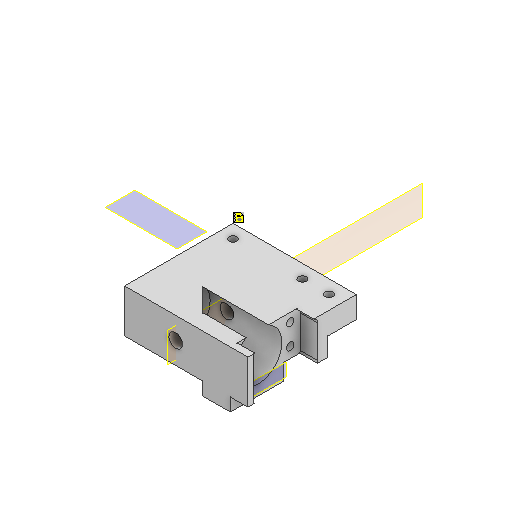
# Autodesk Inventor part: 30_Lightsheet_generator_passive_base_v1
Saved by Autodesk Inventor 2025.3 (Build 293356000, 356)
## iProperties
Created: 2022-12-16
Part Number: 30_Lightsheet_generator_passive_base_v1
Material: Generisch
Document SubType Name: Modeling
Designer: UC2
Density: 1 g/cm^3
Appearance: Vorgabe
Author: UC2
Autodesk Inventor part; units mm, degrees
ref_plane "YZ Plane" through (0, 0, 0) normal (1, 0, 0) x (0, 1, 0)
ref_plane "XZ Plane" through (0, 0, 0) normal (0, 1, 0) x (-1, 0, 0)
ref_plane "XY Plane" through (0, 0, 0) normal (0, 0, 1) x (1, 0, 0)
ref_plane "Arbeitsebene6" through (-62.1, 3.95, -31.1) normal (0, -1, 0) x (1, 0, 0)
sketch "Skizze13" plane through (18.9, 3.95, -31.1) normal (0, 1, 0) x (-1, 0, 0)
  circle A0 centre (40.5, 5) radius 1.45 projected
  line L0 (29.1796, 0.9) -> (29.1796, 0) projected
  line L1 (45.5, 0) -> (29.1796, 0) projected
  line L2 (45.5, 0) -> (45.5, 10) projected
  line L3 (45.5, 10) -> (29.1796, 10) projected
  line L4 (29.1796, 10) -> (29.1796, 6.8717) projected
  line L5 (29.1796, 6.8717) -> (32.9296, 6.8717) projected
  line L6 (32.9296, 6.8717) -> (32.9296, 0.9) projected
  line L7 (32.9296, 0.9) -> (29.1796, 0.9) projected
  line L8 (24.1796, 0) -> (24.1796, 0.9) projected
  line L9 (24.1796, 0.9) -> (20.4296, 0.9) projected
  line L10 (20.4296, 0.9) -> (20.4296, 6.8717) projected
  line L11 (20.4296, 6.8717) -> (24.1796, 6.8717) projected
  line L12 (24.1796, 6.8717) -> (24.1796, 10) projected
  line L13 (24.1796, 10) -> (0, 10) projected
  line L14 (0, 0) -> (0, 10) projected
  line L15 (24.1796, 0) -> (0, 0) projected
  circle A1 centre (14.9199, 5) radius 1.45 projected
  circle A2 centre (5.0801, 5) radius 1.45 projected
  line L16 (29.1796, 10) -> (24.1796, 10)
  line L17 (29.1796, 0) -> (24.1796, 0)
  line L18 (55.5, 0) -> (55.5, 10) projected
  line L19 (55.5, 10) -> (55.473, 10) projected
  line L20 (55.473, 10) -> (55.473, 40) projected
  line L21 (55.473, 40) -> (45.5, 40) projected
  line L22 (45.5, 40) -> (45.5, 20) projected
  line L23 (45.5, 20) -> (35.5, 20) projected
  line L24 (35.5, 20) -> (35.5, 10.0274) projected
  arc A3 (35.5, 10.0274) -> (35.527, 10) centre (40.5, 14.9264) ccw projected
  line L25 (45.5, 10) -> (35.527, 10) projected
  line L26 (45.5, 0) -> (45.5, 10) projected
  line L27 (45.5, 0) -> (55.5, 0) projected
  line L28 (52.073, 16.5) -> (52.073, 3.5) projected
  arc A4 (48.873, 3.5) -> (52.073, 3.5) centre (50.473, 3.5) ccw projected
  line L29 (48.873, 3.5) -> (48.873, 16.5) projected
  arc A5 (52.073, 16.5) -> (48.873, 16.5) centre (50.473, 16.5) ccw projected
  line L30 (48.8865, 23.1111) -> (48.8865, 36.1111) projected
  arc A6 (52.0865, 36.1111) -> (48.8865, 36.1111) centre (50.4865, 36.1111) ccw projected
  line L31 (52.0865, 36.1111) -> (52.0865, 23.1111) projected
  arc A7 (48.8865, 23.1111) -> (52.0865, 23.1111) centre (50.4865, 23.1111) ccw projected
  line L32 (-10, 0) -> (0, 0) projected
  line L33 (0, 10) -> (0, 0) projected
  line L34 (16, 10) -> (0, 10) projected
  line L35 (16, 10) -> (16, 20) projected
  line L36 (16, 20) -> (-10, 20) projected
  line L37 (-10, 20) -> (-10, 0) projected
  line L38 (-3.4, 16.5) -> (-3.4, 3.5) projected
  arc A8 (-6.6, 3.5) -> (-3.4, 3.5) centre (-5, 3.5) ccw projected
  line L39 (-6.6, 3.5) -> (-6.6, 16.5) projected
  arc A9 (-3.4, 16.5) -> (-6.6, 16.5) centre (-5, 16.5) ccw projected
  line L40 (0, 40) -> (45.5, 40)
  line L41 (45.5, 40) -> (45.5, 20.5)
  line L42 (45.5, 20.5) -> (0, 20.5)
  line L43 (0, 20.5) -> (0, 40)
  line L44 (45.5, 20.5) -> (35.5, 20.5)
  line L45 (35.5, 20.5) -> (35.5, 20)
  line L46 (35.5, 20) -> (45.5, 20)
  line L47 (45.5, 20) -> (45.5, 20.5)
  line L48 (16, 20) -> (0, 20)
  line L49 (0, 20) -> (0, 20.5)
  line L50 (0, 20.5) -> (16, 20.5)
  line L51 (16, 20.5) -> (16, 20)
  line L52 (0, 20) -> (0, 10)
  line L53 (35.5, 10) -> (45.5, 10)
  line L54 (45.5, 10) -> (45.5, 20.5)
  line L55 (45.5, 20.5) -> (35.5, 20.5)
  line L56 (35.5, 20.5) -> (35.5, 10)
  line L57 (0, 20.5) -> (-10.5, 20.5)
  line L58 (-10.5, 20.5) -> (-10.5, 0.5)
  line L59 (-10.5, 0.5) -> (0, 0.5)
  line L60 (0, 0.5) -> (0, 20.5)
  point P0 (0, 20)
  point P1 (0.5252, 10)
  point P2 (35.527, 10)
  point P3 (0, 20)
  point P4 (35.5, 10.0274)
  point P5 (-10.5, 20.5)
  dimension "d60" = 0.5
  dimension "d93" = 20
  dimension "d94" = 0.5
  constraints: 47 end point, 11 parallel, 6 horizontal, 6 perpendicular, 2 point on line
  measures "d60" distance between parallel lines of L23 L42
  measures "d93" distance of L57.end L58.end
  measures "d94" distance between parallel lines of L58 L37
extrude "Extrusion12" add sketch "Skizze13" along normal blind 8 contours L7 L6 L5 L4 L3 L2 L1 L0 | L0 L17 L8 L9 L10 L11 L12 L16 L4 L5 L6 L7 | L15 L14 L13 L12 L11 L10 L9 L8 | L3 A3 L24 L23 L54 | L23 L45 L42 L22 | L16 L13 L35 L51 L42 L45 L24 L56 L3 | L42 L43 L40 L22 | L52 L36 L35 L13 | L49 L42 L51 L36
sketch "Skizze16" plane through (18.9, 3.95, -31.1) normal (0, -1, 0) x (1, 0, 0)
  line L0 (-45.5, 0) -> (-45.5, 40) projected
  circle A0 centre (-5.0801, 5) radius 1.45 projected
  circle A1 centre (-14.9199, 5) radius 1.45 projected
  line L1 (-16, 20) -> (10, 20) projected
  line L2 (-66.9798, -10.3003) -> (9.2505, 65.9301)
  line L3 (7.6336, 20.5) -> (0, 20.5) projected
  line L4 (7.6336, 20.5) -> (-54.1544, 20.5)
  line L5 (-54.1544, 20.5) -> (-54.1544, 40)
  line L6 (-54.1544, 40) -> (7.6336, 40)
  line L7 (7.6336, 40) -> (7.6336, 20.5)
  line L8 (-45.5, 40) -> (0, 40) projected
  line L9 (0, 0) -> (-45.5, 0) projected
  line L10 (0, 40) -> (0, 0) projected
  line L11 (0, 40) -> (0, 20.5)
  point P0 (-18.9, 31.1)
  point P1 (-45.5, 20.5)
  point P2 (-45.2879, 40)
  point P3 (10.5, 20.5)
  point P4 (0, 20.5)
  point P5 (0, 40)
  constraints: 12 end point, 2 parallel, 1 horizontal, 1 perpendicular, 1 vertical, 3 other
extrude "Extrusion13" add sketch "Skizze16" along normal blind 8 contours L0 L6 L2 L4 | L2 L6 L10 L4
ref_plane "Arbeitsebene7" through (-7.7796, -1.85, -37.9251) normal (1, 0, 0) x (0, -1, 0)
sketch "Skizze18" plane through (-7.7796, -1.85, -37.9251) normal (1, 0, 0) x (0, -1, 0)
  arc A0 (-5.8, -13.6968) -> (-0.7, -9.8391) centre (-5.8, -8.3968) ccw projected
  line L0 (-0.7, -9.8391) -> (-0.7, -7.7251) projected
  arc A1 (-10.8, -9.8251) -> (-0.8, -9.8251) centre (-5.8, -8.3968) ccw projected
  line L1 (-0.8, -7.8251) -> (-0.8, -9.8251) projected
  line L2 (-10.8, -7.8251) -> (-0.8, -7.8251) projected
  line L3 (-10.8, -9.8251) -> (-10.8, -7.8251) projected
  arc A2 (-10.9, -9.8391) -> (-0.7, -9.8391) centre (-5.8, -8.3968) ccw
  line L4 (-10.9, -9.8391) -> (-10.9, -7.7251)
  line L5 (-10.9, -7.7251) -> (-0.7, -7.7251)
  line L6 (-0.7, -7.7251) -> (-0.7, -9.8391)
  point P0 (-1.85, -37.9251)
  point P1 (-5.8, -13.6968)
  constraints: 6 end point, 2 point on circle, 1 centre point, 3 other
extrude "Extrusion15" cut sketch "Skizze18" along normal mid plane 12.5 contours A2 L4 L5 L0 A0 | L3 L2 L1 A1
ref_plane "Arbeitsebene8" through (22.1204, -2.15, -7.2) normal (1, 0, 0) x (0, 1, 0)
ref_plane "Arbeitsebene9" through (-36.7921, -9.8415, -30.1125) normal (-0.7071068, 0, 0.7071068) x (0.7071068, 0, 0.7071068)
ref_plane "Arbeitsebene10" through (16.1879, 11.05, 2.9992) normal (-1, 0, 0) x (0, 0, 1)
sketch "Skizze21" plane through (16.1879, 11.05, 2.9992) normal (-1, 0, 0) x (0, 0, 1)
  arc A0 (-3.1969, -9.9981) -> (-5.2274, -9.9178) centre (-4.0992, -7.1) ccw projected
  circle A1 centre (-4.0992, -7.1) radius 9
  line L0 (-13.0992, -7.1) -> (4.9008, -7.1)
  line L1 (4.9008, -7.1) -> (4.9008, -20.07)
  line L2 (4.9008, -20.07) -> (-13.0992, -20.07)
  line L3 (-13.0992, -20.07) -> (-13.0992, -7.1)
  point P0 (-2.9992, -11.05)
  dimension "d75" = 18
  constraints: 8 end point, 2 parallel, 2 point on circle, 1 centre point, 1 coincident, 1 horizontal, 1 perpendicular
  measures "d75" diameter of A1
ref_plane "Arbeitsebene11" through (-36.7921, -9.8415, -30.1125) normal (-0.7071068, 0, 0.7071068) x (0.7071068, 0, 0.7071068)
extrude "Extrusion18" cut sketch "Skizze21" along normal up to surface contours L0 A0 | L0 A1 | A0 L0 A1 surface through (-36.7921, -9.8415, -30.1125) normal (-0.7071068, 0, 0.7071068)
sketch "Skizze22" plane through (18.9, -4.05, -31.1) normal (0, -1, 0) x (1, 0, 0)
  line L0 (-34.6684, 23.7083) -> (-19.8191, 38.5575)
  line L1 (-19.8191, 38.5575) -> (-18.9706, 37.709)
  line L2 (-18.9706, 37.709) -> (-33.8198, 22.8597)
  line L3 (-33.8198, 22.8597) -> (-34.6684, 23.7083)
  line L4 (-34.6684, 23.7083) -> (-18.9706, 37.709) construction
  line L5 (-19.8191, 38.5575) -> (-33.8198, 22.8597) construction
  line L6 (-34.6684, 23.7083) -> (-13.6684, 23.7083) construction
  line L7 (-45.5, 40) -> (-45.5, 20.5) projected
  line L8 (0, 40) -> (-45.5, 40) projected
  line L9 (-45.5, 20.5) -> (0, 20.5) projected
  line L10 (0, 20.5) -> (0, 40) projected
  point P0 (-18.9, 31.1)
  point P1 (-26.8195, 30.7086)
  dimension "d78" = 21
  dimension "d79" = 45
  dimension "d80" = 1.2
  constraints: 14 end point, 2 midpoint, 2 parallel, 1 equal length, 1 horizontal, 1 perpendicular
  measures "d78" distance of L0.start L0.end
  measures "d79" angle of L6 L0
  measures "d80" distance of L0.end L1.end
extrude "Extrusion19" cut sketch "Skizze22" against normal blind 14 contours L0 L1 L2 L3
sketch "Skizze23" plane through (18.9, -4.05, -31.1) normal (0, -1, 0) x (1, 0, 0)
  line L0 (-35.6796, 21) -> (-32.9713, 23.7083)
  line L1 (-33.3878, 23.2918) -> (-30.8027, 25.8769) projected
  line L2 (-2.7121, 21) -> (-35.6796, 21) projected
  line L3 (-32.9713, 21) -> (-32.9713, 23.7083)
  line L4 (-18.9706, 37.709) -> (-19.9714, 36.7082) projected
  line L5 (-19.9714, 36.7082) -> (-17.0744, 36.7082)
  line L6 (-17.0744, 36.7082) -> (-17.0744, 39)
  line L7 (-18.9706, 37.709) -> (-33.8198, 22.8597) projected
  line L8 (-19.9714, 36.7082) -> (-17.6796, 39)
  line L9 (-17.6796, 39) -> (-17.0744, 39)
  line L10 (-45.5, 40) -> (-45.5, 20.5) projected
  line L11 (0, 40) -> (-45.5, 40) projected
  line L12 (-45.5, 20.5) -> (0, 20.5) projected
  line L13 (0, 20.5) -> (0, 40) projected
  point P0 (-18.9, 31.1)
  point P1 (-29.1796, 21)
  constraints: 12 end point, 2 horizontal, 2 perpendicular, 2 point on line, 1 collinear
extrude "Extrusion20" add sketch "Skizze23" against normal up to surface (16 mm away) contours L0 L3 L2 | L8 L9 L6 L5 L4
ref_plane "Arbeitsebene12" through (-26.6, -8.85, -11.1) normal (1, 0, 0) x (0, 1, 0)
sketch "Skizze25" plane through (18.9, 3.95, -10.6) normal (1, 0, 0) x (0, 0, -1)
  line L0 (0.5, -6.8) -> (20.5, -6.8) projected
  line L1 (0, -8) -> (0, 8) projected
  line L2 (0, 0) -> (10.5, 0) projected
  line L3 (0, 0) -> (10, 0)
  line L4 (10, 0) -> (10, -6.8)
  line L5 (10, -6.8) -> (0, -6.8)
  line L6 (0, -6.8) -> (0, 0)
  line L7 (10.5, 0) -> (10.5, -6.8) projected
  point P0 (-10.6, -3.95)
  point P1 (0, -6.8)
  dimension "d87" = 0.5
  constraints: 8 end point, 2 parallel, 1 horizontal, 1 perpendicular, 1 point on line
  measures "d87" distance between parallel lines of L7 L4
extrude "Extrusion22" add sketch "Skizze25" against normal up to surface (45.5 mm away) contours L5 L1 L2 L4 L0
sketch "Skizze26" plane through (18.9, 11.95, -31.1) normal (0, 0, -1) x (-1, 0, 0)
  line L0 (0, -8) -> (24.1796, -8) projected
  line L1 (0, 0) -> (24.1796, 0) projected
  line L2 (0, -8) -> (0, 0) projected
  line L3 (24.1796, -8) -> (29.1796, -8) projected
  circle A0 centre (26.6796, -8) radius 2.5
  line L4 (24.1796, -8) -> (24.1796, 0) projected
  point P0 (18.9, -11.95)
  constraints: 1 horizontal alignment, 2 other
extrude "Extrusion23" cut sketch "Skizze26" against normal through all contours A0 L3 | L3 A0
sketch "Skizze30" plane through (-7.7796, -1.85, -37.9251) normal (1, 0, 0) x (0, -1, 0)
  circle A0 centre (-5.8, -38.5222) radius 2.5 projected
  line L0 (-23.3912, -36.8251) -> (18.065, -36.8251)
  circle A1 centre (-5.8, -36.8251) radius 0.9537
  point P0 (-1.85, -37.9251)
  constraints: 2 end point, 1 centre point, 1 horizontal, 1 point on line, 2 other
extrude "Extrusion27" cut sketch "Skizze30" against normal blind 12 contours A1 L0 A0 | A0 A1 | A1 L0 picked at (-5.7305, -36.5604)
sketch "Skizze31" plane through (18.9, 3.95, -31.1) normal (1, 0, 0) x (0, 0, -1)
  arc A0 (-23, -8) -> (-22, -7) centre (-23, -7) ccw projected
  line L0 (-22, 7) -> (-22, -7) projected
  arc A1 (-22, 7) -> (-23, 8) centre (-23, 7) ccw projected
  line L1 (-37, 8) -> (-23, 8) projected
  arc A2 (-37, 8) -> (-38, 7) centre (-37, 7) ccw projected
  line L2 (-38, -7) -> (-38, 7) projected
  arc A3 (-38, -7) -> (-37, -8) centre (-37, -7) ccw projected
  line L3 (-23, -8) -> (-37, -8) projected
  arc A4 (-32.728, 6.725) -> (-34.46, 5.725) centre (-32.728, 4.725) ccw projected
  line L4 (-27.272, 6.725) -> (-32.728, 6.725) projected
  arc A5 (-25.54, 5.725) -> (-27.272, 6.725) centre (-27.272, 4.725) ccw projected
  line L5 (-22.812, 1) -> (-25.54, 5.725) projected
  arc A6 (-22.812, -1) -> (-22.812, 1) centre (-24.544, 0) ccw projected
  line L6 (-25.54, -5.725) -> (-22.812, -1) projected
  arc A7 (-27.272, -6.725) -> (-25.54, -5.725) centre (-27.272, -4.725) ccw projected
  line L7 (-32.728, -6.725) -> (-27.272, -6.725) projected
  arc A8 (-34.46, -5.725) -> (-32.728, -6.725) centre (-32.728, -4.725) ccw projected
  line L8 (-37.188, -1) -> (-34.46, -5.725) projected
  arc A9 (-37.188, 1) -> (-37.188, -1) centre (-35.456, 0) ccw projected
  line L9 (-34.46, 5.725) -> (-37.188, 1) projected
  circle A10 centre (-17.9023, -2.836) radius 1.4 projected
  circle A11 centre (-17.9023, 4.925) radius 1.4 projected
  line L10 (-20.1, -8) -> (-20.1, -6.7) projected
  line L11 (-20.1, -6.7) -> (-14.4396, -6.7) projected
  arc A12 (-14.4396, -6.7) -> (-14.3131, -6) centre (-16.3131, -6) ccw projected
  line L12 (-14.3131, -6) -> (-14.3131, 6) projected
  arc A13 (-14.3131, 6) -> (-16.3131, 8) centre (-16.3131, 6) ccw projected
  line L13 (-16.3131, 8) -> (-23, 8) projected
  arc A14 (-22, 7) -> (-23, 8) centre (-23, 7) ccw projected
  line L14 (-22, -7) -> (-22, 7) projected
  arc A15 (-23, -8) -> (-22, -7) centre (-23, -7) ccw projected
  line L15 (-23, -8) -> (-20.1, -8) projected
  line L16 (-23, 8.1) -> (-16.3131, 8.1)
  arc A16 (-14.2131, 6) -> (-16.3131, 8.1) centre (-16.3131, 6) ccw
  line L17 (-14.2131, 6) -> (-14.2131, -6)
  arc A17 (-14.3715, -6.8) -> (-14.2131, -6) centre (-16.3131, -6) ccw
  line L18 (-14.3715, -6.8) -> (-20, -6.8)
  line L19 (-20, -6.8) -> (-20, -8.1)
  line L20 (-20, -8.1) -> (-23, -8.1)
  line L21 (-23, -8.1) -> (-37, -8.1)
  arc A18 (-38.1, -7) -> (-37, -8.1) centre (-37, -7) ccw
  line L22 (-38.1, -7) -> (-38.1, 7)
  arc A19 (-37, 8.1) -> (-38.1, 7) centre (-37, 7) ccw
  line L23 (-37, 8.1) -> (-23, 8.1)
  point P0 (-31.1, -3.95)
  dimension "d113" = 0.1
  dimension "d114" = 0.1
  constraints: 16 end point, 8 point on circle, 4 centre point, 10 other
  measures "d113" distance between parallel lines of L11 L18
  measures "d114" distance between parallel lines of L3 L21
ref_plane "Arbeitsebene13" through (12.4, -4.05, -16.7869) normal (-1, 0, 0) x (0, 0, 1)
extrude "Extrusion28" cut sketch "Skizze31" against normal up to surface (6.5 mm away) contours L3 A3 L2 A2 L1 A1 L0 A0 | A0 L0 A1 L13 A13 L12 A12 L11 L10 L15 | L4 A5 L5 A6 L6 A7 L7 A8 L8 A9 L9 A4 | A10 | A11 | L16 A16 L17 A17 L18 L19 L20 L21 A18 L22 A19 L23
sketch "Skizze32" plane through (12.4, -2.05, -16.7869) normal (1, 0, 0) x (0, 0, -1)
  circle A0 centre (-3.5892, 3.164) radius 1.4 projected
  circle A1 centre (-3.5892, 10.925) radius 1.4 projected
  point P0 (-16.7869, 2.05)
extrude "Extrusion29" cut sketch "Skizze32" against normal blind 10
sketch "Skizze33" plane through (12.4, -3.05, 7) normal (1, 0, 0) x (0, 0, -1)
  line L0 (38.1, -5.8) -> (18.1, -5.8) projected
  line L1 (38.1, -5.8) -> (38.1, 0.2) projected
  line L2 (18.1, 0.2) -> (38.1, 0.2) projected
  line L3 (18.1, -5.8) -> (18.1, 0.2) projected
  line L4 (15.1, -1) -> (18, -1) projected
  line L5 (0.6417, -1) -> (-1.9, -1) projected
  line L6 (17.6, 0.2) -> (17.6, -1) projected
  line L7 (15.1, -1) -> (1.1, -1) projected
  arc A0 (12.2231, -1) -> (12.2231, 15) centre (8.1, 7) ccw projected
  circle A1 centre (8.1, 7) radius 9
  line L8 (17.6, -1) -> (17.6, -5.8)
  line L9 (17.6, -5.8) -> (-1.9, -5.8)
  line L10 (-1.9, -5.8) -> (-1.9, -1)
  line L11 (-1.9, -1) -> (17.6, -1) projected
  line L12 (3.9769, -1) -> (-1.9, -1)
  point P0 (7, 3.05)
  point P1 (3.9769, -1)
  constraints: 8 end point, 2 perpendicular, 2 point on circle, 1 centre point, 1 coincident, 1 horizontal, 1 point on line, 1 vertical
ref_plane "Arbeitsebene14" through (-36.7921, -9.8415, -30.1125) normal (-0.7071068, 0, 0.7071068) x (0.7071068, 0, 0.7071068)
extrude "Extrusion30" add sketch "Skizze33" against normal up to surface contours L4 L8 L9 L10 L5 L11 L7 A1 surface through (-36.7921, -9.8415, -30.1125) normal (-0.7071068, 0, 0.7071068)
sketch "Skizze34" plane through (12.4, -8.85, -10.6) normal (0, -1, 0) x (1, 0, 0)
  line L0 (-12.4706, 17.209) -> (-13.4714, 16.2082) projected
  line L1 (-13.3191, 18.0575) -> (-12.4706, 17.209) projected
  line L2 (-28.1684, 3.2083) -> (-13.3191, 18.0575) projected
  line L3 (-27.3198, 2.3597) -> (-28.1684, 3.2083) projected
  line L4 (-26.4713, 3.2083) -> (-27.3198, 2.3597) projected
  line L5 (-13.4714, 16.2082) -> (-26.4713, 3.2083) projected
  line L6 (-13.3191, 18.4897) -> (-12.0384, 17.209)
  line L7 (-12.0384, 17.209) -> (-13.2553, 15.9921)
  line L8 (-13.2553, 15.9921) -> (-26.2552, 2.9922)
  line L9 (-26.2552, 2.9922) -> (-27.3198, 1.9276)
  line L10 (-27.3198, 1.9276) -> (-28.6005, 3.2083)
  line L11 (-28.6005, 3.2083) -> (-13.3191, 18.4897)
  point P0 (-12.4, 10.6)
  constraints: 12 end point, 5 other
extrude "Extrusion31" cut sketch "Skizze34" against normal blind 10 contours L0 L5 L4 L3 L2 L1 | L6 L7 L8 L9 L10 L11
sketch "Skizze35" plane through (12.4, -2.05, -16.8869) normal (1, 0, 0) x (0, 0, -1)
  circle A0 centre (-3.6892, 3.164) radius 1.4 projected
  circle A1 centre (-3.6892, 10.925) radius 1.4 projected
  arc A2 (-23.8869, 2.077) -> (-11.6638, 14) centre (-15.7869, 6) ccw projected
  line L0 (-23.8869, 2.077) -> (-23.8869, -1) projected
  arc A3 (-23.8869, -1) -> (-23.2452, -2) centre (-22.7869, -1) ccw projected
  line L1 (-25.7869, -2) -> (-23.2452, -2) projected
  line L2 (-25.7869, -2) -> (-25.7869, -6.8) projected
  line L3 (-25.7869, -6.8) -> (-6.2869, -6.8) projected
  line L4 (-6.2869, -0.8) -> (-6.2869, -6.8) projected
  line L5 (-0.1584, -0.8) -> (-6.2869, -0.8) projected
  arc A4 (-0.1584, -0.8) -> (0, 0) centre (-2.1, 0) ccw projected
  line L6 (0, 0) -> (0, 12) projected
  arc A5 (0, 12) -> (-1.4597, 14) centre (-2.1, 12) ccw projected
  line L7 (-11.6638, 14) -> (-1.4597, 14) projected
  arc A6 (-23.8869, -1) -> (-23.2452, -2) centre (-22.7869, -1) ccw projected
  line L8 (-23.8869, -1) -> (-23.8869, 13) projected
  arc A7 (-23.2452, 14) -> (-23.8869, 13) centre (-22.7869, 13) ccw projected
  line L9 (-25.7869, 14) -> (-23.2452, 14) projected
  line L10 (-25.7869, 14) -> (-25.7869, -2) projected
  line L11 (-23.2452, -2) -> (-25.7869, -2) projected
  circle A8 centre (-15.7869, 6) radius 3
  line L12 (-20.5369, 10.75) -> (-11.0369, 10.75) construction
  line L13 (-11.0369, 10.75) -> (-11.0369, 1.25) construction
  line L14 (-11.0369, 1.25) -> (-20.5369, 1.25) construction
  line L15 (-20.5369, 1.25) -> (-20.5369, 10.75) construction
  line L16 (-20.5369, 10.75) -> (-11.0369, 1.25) construction
  line L17 (-11.0369, 10.75) -> (-20.5369, 1.25) construction
  circle A9 centre (-11.0369, 1.25) radius 1
  circle A10 centre (-20.5369, 1.25) radius 1
  circle A11 centre (-20.5369, 10.75) radius 1
  circle A12 centre (-11.0369, 10.75) radius 1.25
  line L18 (-11.6638, 14) -> (-23.2452, 14)
  point P0 (-16.8869, 2.05)
  point P1 (-25.7869, -2)
  dimension "d120" = 6
  dimension "d121" = 9.5
  dimension "d122" = 9.5
  dimension "d123" = 2
  dimension "d124" = 2
  dimension "d125" = 2
  dimension "d126" = 2.5
  constraints: 14 end point, 5 centre point, 5 coincident, 2 horizontal, 2 midpoint, 2 parallel, 1 perpendicular
  measures "d120" diameter of A8
  measures "d121" distance of L13.end L14.end
  measures "d122" distance of L12.end L13.end
  measures "d123" diameter of A9
  measures "d124" diameter of A10
  measures "d125" diameter of A11
  measures "d126" diameter of A12
ref_plane "Arbeitsebene15" through (25.4, -2.775, -8.556) normal (1, 0, 0) x (0, 1, 0)
extrude "Extrusion32" [suppressed]
